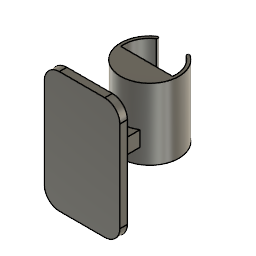
Motor Support (Autodesk Fusion 360 design; units mm, degrees)
Autodesk Fusion 360 part; units mm, degrees
sketch "Sketch1" plane through (0, 0, 0) normal (0, 0, 1) x (1, 0, 0)
  line L0 (0, 0) -> (50, 0)
  line L1 (50, 0) -> (50, 5)
  line L2 (50, 5) -> (0, 5)
  line L3 (0, 5) -> (0, 0)
  circle A0 centre (25, 44.774) radius 19.25
  line L4 (25, 147.1554) -> (25, 0)
  circle A1 centre (25, 44.774) radius 17.25
  line L5 (15, 5) -> (15, 28.3252)
  line L6 (35, 5) -> (35, 28.3252)
  line L7 (14.2966, 60.774) -> (35.7034, 60.774)
  line L8 (5.776, 43.774) -> (44.224, 43.774)
  point P0 (25, 5)
  point P1 (25, 27.524)
  dimension "d1" = -2
  dimension "d2" = 34.5
  dimension "d3" = 50
  dimension "d4" = 27.524
  dimension "d5" = 5
  dimension "d6" = 20
  dimension "d19" = 16
  dimension "d24" = 1
  constraint horizontal L0
  constraint vertical L1
  constraint horizontal L2
  constraint vertical L3
  constraint coincident L0.start L3.end
  constraint coincident A0.centre L4
  constraint midpoint L2 P0
  constraint midpoint L0 L4.end
  constraint vertical L4
  constraint coincident L2 L5.start
  constraint coincident A0 L5.end
  constraint perpendicular L2 L5
  constraint coincident L2 L6.start
  constraint coincident A0 L6.end
  constraint perpendicular L2 L6
  constraint coincident A1 P1
  constraint coincident L4 P1
  constraint symmetric L4 L5 L6
  constraint coincident A0 L7.start
  constraint coincident A0 L7.end
  constraint horizontal L7
  constraint coincident A0 L8.start
  constraint coincident A0 L8.end
  constraint perpendicular L4 L8
  measures "d2" diameter of A1
  measures "d3" distance of L1 L3
  measures "d4" distance of L4.end P1
  measures "d5" distance of L0 L2
  measures "d6" distance of L5 L6
  measures "d19" distance of A0.centre L7
  measures "d24" distance of A0.centre L8
extrude "Extrude1" add sketch "Sketch1" along normal blind 30 and the other way blind 15 contours A0 L4 A1 L8 | A0 L4 A1 L8 | A0 A1 L7 L8 | A0 A1 L7 L8
extrude "Extrude2" add sketch "Sketch1" along normal mid plane 10 contours L2 A0 L4 L6 | L2 A0 L4 L5
extrude "Extrude3" add sketch "Sketch1" along normal mid plane 80 contours L0 L2 L3 L4 | L0 L1 L2 L4
fillet "Fillet1" radius 10 4 edges at (0, 2.5, -40) (0, 2.5, 40) (50, 2.5, 40) (50, 2.5, -40)
fillet "Fillet3" radius 10 2 edges at (25, 5, -5) (25, 5, 5)
extrude "Extrude4" add sketch "Sketch1" along normal blind 2 from surface at 30 contours A0 L4 A1 L8 | A0 L4 A1 L8 | L4 A1 L8 | L4 A1 L8 | A0 A1 L7 L8 | A0 A1 L7 L8
fillet "Fillet4" radius 1 4 edges at (14.2966, 60.774, 8.5) (18.5531, 60.774, 8.5) (31.4469, 60.774, 8.5) (35.7034, 60.774, 8.5)
fillet "Fillet4" radius 1 2 edges at (25, 43.774, 32) (25, 43.774, 30)
